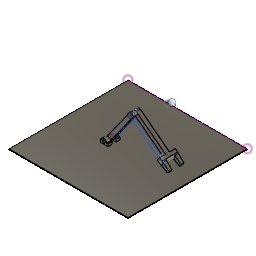
5746c2d5-004e-4e03-9d9f-65d65858cfc3 (Autodesk Fusion 360 design; units mm, degrees)
Autodesk Fusion 360 part; units mm, degrees
note: some values were not read from the file. Chosen so that the rebuilt part matches the saved one: which bodies a step acts on. Set by a fixed rule: which sketch regions a step uses.
sketch "Sketch2" plane through (0, 0, 0) normal (0, 0, 1) x (1, 0, 0)
  line L0 (0, 0) -> (-300, 0)
  line L1 (-300, 0) -> (-300, -300)
  line L2 (-300, -300) -> (0, -300)
  line L3 (0, -300) -> (0, 0)
  dimension "d1" = 300
  dimension "d2" = 300
  dimension "d59" = 0
  dimension "d60" = 0
  dimension "d61" = 0
  dimension "d62" = 0
extrude "Extrude1" add sketch "Sketch2" along normal blind 2 makes body 1
sketch "Sketch3" plane through (0, 0, 0) normal (0, 1, 0) x (1, 0, 0)
  line L0 (0, -2) -> (-300, -2)
  line L1 (-199.6936, -2) -> (-179.6936, -2)
  line L2 (-179.6936, -2) -> (-179.6936, -8)
  line L3 (-199.6936, -2) -> (-199.6936, -7.9996)
  line L4 (-199.6936, -7.9996) -> (-195.6936, -7.9996)
  line L5 (-179.6936, -8) -> (-183.6936, -8)
  arc A0 (-195.6936, -7.9996) -> (-183.6936, -8) centre (-189.6936, -8.0113) ccw
  circle A1 centre (-189.6936, -8.0113) radius 3
  dimension "d5" = 20
  dimension "d6" = 6
  dimension "d7" = 4
  dimension "d8" = 4
  dimension "d9" = 6
  measures "d9" diameter of A1
extrude "Extrude2" add sketch "Sketch3" along normal blind 10 from surface at -150 bodies 1
extrude "Extrude3" add sketch "Sketch3" along normal blind 10 from surface at -170 bodies 1
sketch "Sketch4" plane through (0, -150, 0) normal (0, -1, 0) x (1, 0, 0)
  circle A0 centre (-189.6936, 8.0113) radius 3
  line L0 (-199.6936, 7.9996) -> (-199.6936, 2)
  line L1 (-199.6936, 2) -> (-179.6936, 2)
  line L2 (-179.6936, 2) -> (-179.6936, 8)
  line L3 (-179.6936, 8) -> (-183.6936, 8)
  arc A1 (-183.6936, 8) -> (-195.6936, 7.9996) centre (-189.6936, 8.0113) ccw
  line L4 (-195.6936, 7.9996) -> (-199.6936, 7.9996)
  arc A2 (-193.774, 10.901) -> (-185.6132, 5.1216) centre (-189.6936, 8.0113) ccw
  line L5 (-189.6936, 8.0113) -> (-193.774, 10.901) construction
  line L6 (-189.6936, 8.0113) -> (-185.6132, 5.1216) construction
  line L7 (-185.6132, 5.1216) -> (-127.8195, 86.7297)
  line L8 (-193.774, 10.901) -> (-135.9803, 92.5091)
  arc A3 (-127.8195, 86.7297) -> (-135.9803, 92.5091) centre (-131.8999, 89.6194) ccw
  dimension "d16" = 5
  dimension "d17" = 180
  dimension "d18" = 100
  dimension "d19" = 100
  measures "d16" radius of A2
  measures "d17" angle of L5 L6
  measures "d18" distance of origin
  measures "d19" distance of origin
extrude "Extrude4" add sketch "Sketch4" along normal up to surface (10 mm away) contours L3 A1 L7 L8 A3 | L3 A1 A2 L7 L8 bodies 1
sketch "Sketch5" plane through (0, -160, 0) normal (0, -1, 0) x (1, 0, 0)
  line L0 (-183.6936, 8) -> (-183.5747, 8)
  line L1 (-183.5747, 8) -> (-127.8195, 86.7297)
  arc A0 (-127.8195, 86.7297) -> (-135.9803, 92.5091) centre (-131.8999, 89.6194) ccw
  line L2 (-135.9803, 92.5091) -> (-191.8572, 13.6076)
  arc A1 (-183.6936, 8) -> (-191.8572, 13.6076) centre (-189.6936, 8.0113) ccw
  circle A2 centre (-131.8999, 89.6194) radius 3
  line L3 (-131.8999, 89.6194) -> (-129.0102, 93.6998)
  line L4 (-131.8999, 89.6194) -> (-134.7896, 85.539)
  line L5 (-129.0102, 93.6998) -> (-49.6501, 32.856)
  line L6 (-134.7896, 85.539) -> (-55.4294, 24.6952)
  arc A3 (-129.0102, 93.6998) -> (-134.7896, 85.539) centre (-131.8999, 89.6194) ccw
  arc A4 (-55.4294, 24.6952) -> (-49.6501, 32.856) centre (-52.3851, 28.6661) ccw
  dimension "d22" = 6
  dimension "d23" = 5
  dimension "d24" = 100
  dimension "d25" = 100
  measures "d22" diameter of A2
extrude "Extrude5" add sketch "Sketch5" against normal up to surface (10 mm away) separate body contours L1 A0 L5 L6 A4 | L1 A0 A2 L3 L4 L6 | A0 A2 L3 L4 A3 makes body 2
extrude "Extrude6" cut sketch "Sketch5" against normal up to surface (10 mm away) contours A2 L3 L4 | A2 L3 L4 bodies 1
sketch "Sketch6" plane through (0, -150, 0) normal (0, 1, 0) x (-1, 0, 0)
  circle A0 centre (131.8999, 89.6194) radius 3
  line L0 (55.4294, 24.6952) -> (134.7896, 85.539)
  arc A1 (134.7896, 85.539) -> (129.0102, 93.6998) centre (131.8999, 89.6194) ccw
  line L1 (129.0102, 93.6998) -> (49.6501, 32.856)
  arc A2 (49.6501, 32.856) -> (55.4294, 24.6952) centre (52.3851, 28.6661) ccw
  line L2 (55.4432, 37.2975) -> (61.5275, 29.3614)
  dimension "d30" = 10
extrude "Extrude7" add sketch "Sketch6" along normal blind 15 contours L0 L1 A2 L2 bodies 2
extrude "Extrude8" add sketch "Sketch6" against normal blind 15 from surface at -10 contours L0 L1 A2 L2 bodies 2
sketch "Sketch7" plane through (-52.9276, 0, 40.5785) normal (-0.793601, 0, 0.608438) x (0, -1, 0)
  line L0 (160, -4.1344) -> (160, -14.1273)
  line L1 (160, -14.1273) -> (175, -14.1273)
  line L2 (175, -14.1273) -> (175, -4.1344)
  line L3 (175, -4.1344) -> (160, -4.1344)
  line L4 (175, -4.1344) -> (175, -14.1344)
  line L5 (175, -14.1344) -> (165, -14.1344)
  line L6 (165, -14.1344) -> (164.971, -4.1344)
  line L7 (175, -4.1344) -> (165, -4.1634)
  line L8 (135, -14.1273) -> (145, -14.1273)
  line L9 (145, -14.1273) -> (145, -4.1273)
  line L10 (145, -4.1273) -> (135, -4.1273)
  line L11 (135, -4.1273) -> (135, -14.1273)
  dimension "d36" = 10
  dimension "d37" = 10
  dimension "d38" = 10
  dimension "d39" = 10
  dimension "d40" = 10
extrude "Extrude9" add sketch "Sketch7" against normal blind 30 draft -3 contours L1 L2 L3 L4 L6 | L8 L9 L10 L11 bodies 2
split "Split1" by plane through (0, 0, 2) normal (0, 0, 1) bodies 1 makes body 3 at (-164.9897, -156.6667, 34.2432)
split "Split2" by plane through (0, -160, 0) normal (0, 1, 0) bodies 3 makes body 4 at (-164.9897, -156.6667, 34.2432)
split "Split3" by plane through (0, -150, 0) normal (0, -1, 0) bodies 4 makes body 5 at (-164.9897, -156.6667, 34.2432)
copy_body "Body->Comp1" bodies 1 removing the originals makes body 6 in component "Component"
copy_body "Body->Comp2" bodies 5 removing the originals makes body 7 in component "Component'"
copy_body "Body->Comp3" bodies 3 removing the originals makes body 8 in component "Component''"
copy_body "Body->Comp4" bodies 4 removing the originals makes body 9 in component "Component'''"
copy_body "Body->Comp5" bodies 2 removing the originals makes body 10 in component "Component''''"
component "Component" placed x (1, 0, 0) y (0, 1, 0) z (0, 0, 1) at (0.3064, 0, 0)
component "Component'" placed x (1, 0, 0) y (0, 1, 0) z (0, 0, 1) at (0.0804, 0, 0.1103)
component "Component''" placed x (1, 0, 0) y (0, 1, 0) z (0, 0, 1) at (0, 0, 0)
component "Component'''" placed x (1, 0, 0) y (0, 1, 0) z (0, 0, 1) at (0, 0, 0)
component "Component''''" placed x (1, 0, 0) y (0, 1, 0) z (0, 0, 1) at (0, 10, 0)
